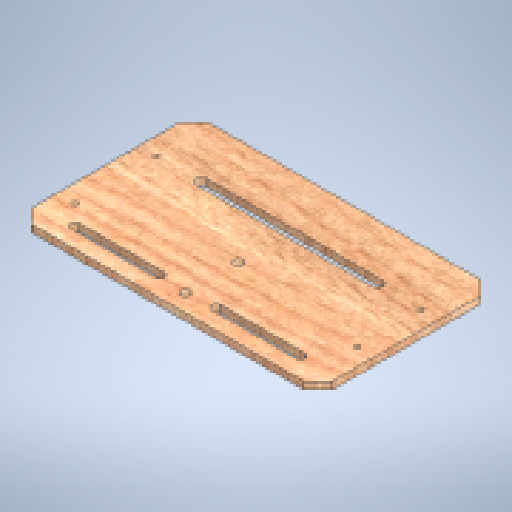
# Autodesk Inventor part: фанера
Saved by Autodesk Inventor 2023.1 (Build 271208000, 208)
## iProperties
Created: 2025-12-23
Part Number: фанера
Material: Древесина (береза)
Document SubType Name: Modeling
Designer: DELL
Density: 0.55 g/cm^3
Appearance: Береза — натуральный — полированный
Author: DELL
Autodesk Inventor part; units mm, degrees
ref_plane "YZ Plane" through (0, 0, 0) normal (1, 0, 0) x (0, 1, 0)
ref_plane "XZ Plane" through (0, 0, 0) normal (0, 1, 0) x (-1, 0, 0)
ref_plane "XY Plane" through (0, 0, 0) normal (0, 0, 1) x (1, 0, 0)
sketch "Эскиз1" plane through (0, 0, 0) normal (0, 1, 0) x (-1, 0, 0)
  line L0 (85.25, 50) -> (-85.25, 50)
  line L1 (-85.25, 50) -> (-85.25, -50)
  line L2 (-85.25, -50) -> (85.25, -50)
  line L3 (85.25, -50) -> (85.25, 50)
  line L4 (85.25, 50) -> (-85.25, -50) construction
  line L5 (-85.25, 50) -> (85.25, -50) construction
  point P0 (0, 0)
  dimension "d0" = 170.5
  dimension "d1" = 100
  constraints: 12 end point, 2 midpoint, 2 parallel, 1 horizontal, 1 perpendicular
  measures "d0" distance of L2.end L1.end
  measures "d1" distance of L1.end L0.end
extrude "Выдавливание1" add sketch "Эскиз1" along normal blind 4
sketch "Эскиз2" plane through (0, 4, 0) normal (0, 1, 0) x (1, 0, 0)
  circle A0 centre (75.25, -18) radius 1.6 projected
  circle A1 centre (-75.25, 18.7) radius 1.6 projected
  circle A2 centre (75.25, 18.2) radius 1.6 projected
  circle A3 centre (-75.25, -27.5) radius 1.6 projected
  point P0 (0, 0)
extrude "Выдавливание2" cut sketch "Эскиз2" against normal blind 4
chamfer "Фаска1" distance 8 angle 45 4 edges at (-85.25, 2, -50) (-85.25, 2, 50) (85.25, 2, -50) (85.25, 2, 50)
sketch "Эскиз3" plane through (0, 4, 0) normal (0, 1, 0) x (1, 0, 0)
  circle A0 centre (0, -40) radius 2.55
  circle A1 centre (0, -10) radius 2.55
  line L0 (-85.25, 42) -> (-85.25, -42) projected
  line L1 (-77.25, -50) -> (77.25, -50) projected
  point P0 (0, 0)
  dimension "d11" = 85.25
  dimension "d12" = 10
  dimension "d13" = 5.1
  constraints: 2 centre point
  measures "d11" distance from line of L0 A0.centre
  measures "d12" distance from line of L1 A0.centre
  measures "d13" diameter of A0
extrude "Выдавливание3" cut sketch "Эскиз3" against normal blind 10
sketch "Эскиз4" plane through (0, 4, 0) normal (0, 1, 0) x (1, 0, 0)
  circle A0 centre (0, -40) radius 2.55 construction
  line L0 (64, -38.5) -> (16, -38.5) construction
  line L1 (64, -36) -> (16, -36)
  line L2 (16, -41) -> (64, -41)
  arc A1 (64, -41) -> (64, -36) centre (64, -38.5) ccw
  arc A2 (16, -36) -> (16, -41) centre (16, -38.5) ccw
  line L3 (-77.25, -50) -> (77.25, -50) construction
  line L4 (0, -50) -> (0, 0) construction
  line L5 (50, 19) -> (-50, 19) construction
  line L6 (50, 22) -> (-50, 22)
  line L7 (-50, 16) -> (50, 16)
  arc A3 (50, 16) -> (50, 22) centre (50, 19) ccw
  arc A4 (-50, 22) -> (-50, 16) centre (-50, 19) ccw
  line L8 (0, 0) -> (0, 38) construction
  line L9 (-64, -38.5) -> (-16, -38.5) construction
  line L10 (-64, -36) -> (-16, -36)
  line L11 (-16, -41) -> (-64, -41)
  arc A5 (-64, -36) -> (-64, -41) centre (-64, -38.5) ccw
  arc A6 (-16, -41) -> (-16, -36) centre (-16, -38.5) ccw
  line L12 (77.25, -50) -> (-77.25, -50) construction
  point P0 (40, -38.5)
  point P1 (0, 19)
  point P2 (0, 19)
  point P3 (-40, -38.5)
  dimension "d14" = 24
  dimension "d15" = 5
  dimension "d16" = 16
  dimension "d17" = 50
  dimension "d18" = 6
  dimension "d21" = 16
  constraints: 30 end point, 12 point on circle, 9 symmetric about line, 8 tangent, 6 centre point, 4 midpoint, 2 horizontal, 2 parallel, 2 vertical, 1 coincident, 2 other
  measures "d14" distance of point (40, -38.5) L0.end
  measures "d15" diameter of A2
  measures "d16" horizontal distance of L4.end L1.end
  measures "d17" distance of point (0, 19) L5.end
  measures "d18" diameter of A4
  measures "d21" distance from line of L4.end L7
extrude "Выдавливание4" cut sketch "Эскиз4" against normal blind 10
